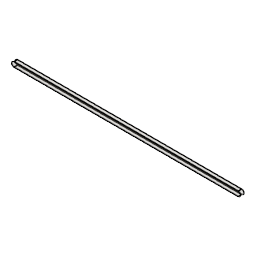
Dado Connection (Autodesk Fusion 360 design; units mm, degrees)
Autodesk Fusion 360 part; units mm, degrees
sketch "Connection Patch" plane through (0, 0, 0) normal (0, 0, 1) x (-1, 0, 0)
  line L0 (-300, 9) -> (300, 9)
  line L1 (300, 9) -> (300, -9)
  line L2 (300, -9) -> (-300, -9)
  line L3 (-300, -9) -> (-300, 9)
  line L4 (-300, 9) -> (300, -9) construction
  line L5 (300, 9) -> (-300, -9) construction
  dimension "d3" = 600
  dimension "d4" = 18
  constraint horizontal L0
  constraint perpendicular L0 L1
  constraint parallel L0 L2
  constraint parallel L1 L3
  constraint coincident L4 origin
  constraint coincident L5 origin
  measures "d3" distance of L1.end L2.end
  measures "d4" distance of L0.end L1.end
sketch "Dado Profile" plane through (0, 0, 0) normal (0, 0, 1) x (-1, 0, 0)
  line L0 (-280, -6) -> (280, -6)
  arc A0 (280, -6) -> (280, 6) centre (280, 0) ccw
  line L1 (280, 6) -> (-280, 6)
  arc A1 (-280, 6) -> (-280, -6) centre (-280, 0) ccw
  line L2 (-280, 0) -> (280, 0) construction
  line L3 (-300, 0) -> (300, 0)
  line L4 (300, -9) -> (-300, -9) construction
  line L5 (-300, -9) -> (-300, 9) construction
  line L6 (300, 9) -> (300, -9) construction
  point P0 (300, 0)
  point P1 (-300, 0)
  dimension "d25" = 3
  dimension "d26" = 20
  dimension "d27" = 20
  constraint tangent L0 A0
  constraint tangent A0 L1
  constraint parallel L0 L1
  constraint tangent L1 A1
  constraint tangent L0 A1
  constraint horizontal L2
  constraint coincident L2 origin
  measures "d25" distance of L0 L4
  measures "d26" distance of A1.centre L5
  measures "d27" distance of A0.centre L6
extrude "Extrude1" add sketch "Dado Profile" along normal blind 9 makes body 1
sketch "Sketch3" plane through (0, 0, 0) normal (0, 0, 1) x (-1, 0, 0)
  arc A0 (-280, 6) -> (-280, -6) centre (-280, 0) ccw
  line L0 (-280, -6) -> (280, -6)
  arc A1 (280, -6) -> (280, 6) centre (280, 0) ccw
  line L1 (280, 6) -> (-280, 6)
  line L2 (280, 5.8) -> (-280, 5.8)
  arc A2 (-280, 5.8) -> (-280, -5.8) centre (-280, 0) ccw
  line L3 (-280, -5.8) -> (280, -5.8)
  arc A3 (280, -5.8) -> (280, 5.8) centre (280, 0) ccw
extrude "Extrude2" add sketch "Sketch3" along normal up to surface (9 mm away) separate body contours L2 A2 L3 A3 makes body 2
move_face "OffsetFaces3" offset -1 1 faces at (-93.3333, 1.9333, 9) on bodies 2
move_face "OffsetFaces4" offset 1 1 faces at (-93.3333, 1.9333, 0) on bodies 2
equation "Length = 600 mm"
equation "Width = 18 mm"
equation "d3 = Length"
equation "d4 = Width"
equation "UserOffset1 = 20 mm"
equation "UserOffset2 = 20 mm"
equation "Offset1 = if(UserOffset1 < 5 mm; 5 mm; UserOffset1)"
equation "Offset2 = if(UserOffset2 < 5 mm; 5 mm; UserOffset2)"
equation "OffsetFromTopBottom = 3 mm"
equation "NestledBoardT = 18 mm"
equation "d14 = NestledBoardT / 2"
equation "GapBetweenMortiseandTenon = 0.2 mm"
equation "GapFromBottom = 1 mm"
equation "d23 = -GapFromBottom"
equation "d25 = OffsetFromTopBottom"
equation "d26 = Offset2"
equation "d27 = Offset1"
equation "d28 = -GapBetweenMortiseandTenon"
named bodies: "Mortise", "Tenon"
